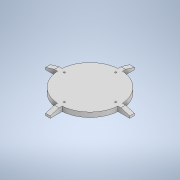
# Autodesk Inventor part: BASE
Saved by Autodesk Inventor 2021 (Build 250183000, 183)
## iProperties
Created: 2023-04-04
Part Number: BASE
Material: Generic
Document SubType Name: Modeling
Designer: PC
Density: 1 g/cm^3
Appearance: Default
Author: PC
Autodesk Inventor part; units mm, degrees
ref_plane "YZ Plane" through (0, 0, 0) normal (1, 0, 0) x (0, 1, 0)
ref_plane "XZ Plane" through (0, 0, 0) normal (0, 1, 0) x (-1, 0, 0)
ref_plane "XY Plane" through (0, 0, 0) normal (0, 0, 1) x (1, 0, 0)
ref_plane "Work Plane17" through (0, -15, 0) normal (0, -1, 0) x (1, 0, 0)
sketch "Sketch131" plane through (0, -15, 0) normal (0, -1, 0) x (1, 0, 0)
  circle A0 centre (0, 0) radius 2.55 projected
  circle A1 centre (0, 0) radius 65
  dimension "d245" = 130
  constraints: 1 centre point, 1 coincident
  measures "d245" diameter of A1
extrude "Extrusion62" add sketch "Sketch131" against normal blind 10 contours A0 | A1
sketch "Sketch132" plane through (0, -15, 0) normal (0, -1, 0) x (1, 0, 0)
  line L0 (5, 40) -> (-5, 40)
  line L1 (-5, 40) -> (-5, 90)
  line L2 (-5, 90) -> (5, 90)
  line L3 (5, 90) -> (5, 40)
  circle A0 centre (0, 0) radius 65 projected
  line L4 (5, 40) -> (-5, 90) construction
  line L5 (-5, 40) -> (5, 90) construction
  line L6 (-40, -5) -> (-90, -5)
  line L7 (-90, -5) -> (-90, 5)
  line L8 (-90, 5) -> (-40, 5)
  line L9 (-40, 5) -> (-40, -5)
  line L10 (-40, -5) -> (-90, 5) construction
  line L11 (-90, -5) -> (-40, 5) construction
  line L12 (5, -40) -> (-5, -40)
  line L13 (-5, -40) -> (-5, -90)
  line L14 (-5, -90) -> (5, -90)
  line L15 (5, -90) -> (5, -40)
  line L16 (5, -40) -> (-5, -90) construction
  line L17 (-5, -40) -> (5, -90) construction
  line L18 (89.9938, -5) -> (39.9938, -5)
  line L19 (39.9938, -5) -> (39.9938, 5)
  line L20 (39.9938, 5) -> (89.9938, 5)
  line L21 (89.9938, 5) -> (89.9938, -5)
  line L22 (89.9938, -5) -> (39.9938, 5) construction
  line L23 (39.9938, -5) -> (89.9938, 5) construction
  point P0 (0, 65)
  point P1 (-65, 0)
  point P2 (0, -65)
  point P3 (64.9938, 0)
  dimension "d248" = 10
  dimension "d249" = 50
  dimension "d250" = 50
  dimension "d251" = 10
  dimension "d252" = 10
  dimension "d253" = 50
  dimension "d254" = 50
  dimension "d255" = 10
  constraints: 48 end point, 8 midpoint, 8 parallel, 4 horizontal, 4 perpendicular, 3 point on circle
  measures "d248" distance of L1.end L2.end
  measures "d249" distance of L0.end L1.end
  measures "d250" distance of L7.end L8.end
  measures "d251" distance of L6.end L7.end
  measures "d252" distance of L14.end L13.end
  measures "d253" distance of L13.end L12.end
  measures "d254" distance of L19.end L20.end
  measures "d255" distance of L18.end L19.end
extrude "Extrusion63" add sketch "Sketch132" against normal blind 10 contours L0 L1 A0 L3 | A0 L1 L2 L3 | L20 L21 L18 A0 | A0 L18 L19 L20 | L8 L9 L6 A0 | A0 L6 L7 L8 | L13 L12 L15 A0 | A0 L15 L14 L13
chamfer "Chamfer1" distance 18.75 distance2 5.5 1 edges at (-90, -5, 0) measured on face at (-89.5, -5, 0)
chamfer "Chamfer2" distance 18.75 distance2 5.5 1 edges at (0, -5, -90) measured on face at (0, -5, -89.5)
chamfer "Chamfer3" distance 18.75 distance2 5.5 1 edges at (89.9938, -5, 0) measured on face at (89.4938, -5, 0)
chamfer "Chamfer4" distance 18.75 distance2 5.5 1 edges at (0, -5, 90) measured on face at (0, -5, 89.5)
sketch "Sketch135" plane through (0, -5, 0) normal (0, 1, 0) x (1, 0, 0)
  circle A0 centre (0, 0) radius 55.054
  circle A1 centre (-55.054, 0) radius 1.55
  circle A2 centre (0, 55.054) radius 1.55
  circle A3 centre (55.054, 0) radius 1.55
  circle A4 centre (0, -55.054) radius 1.55
  dimension "d279" = 110.108
  dimension "d280" = 3.1
  dimension "d281" = 3.1
  dimension "d282" = 3.1
  dimension "d283" = 3.1
  constraints: 5 centre point, 4 point on circle, 1 coincident
  measures "d279" diameter of A0
  measures "d280" diameter of A1
  measures "d281" diameter of A2
  measures "d282" diameter of A3
  measures "d283" diameter of A4
extrude "Extrusion64" cut sketch "Sketch135" against normal blind 30 contours A0 A3 | A0 A3 | A2 A0 | A0 A2 | A4 A0 | A0 A4 | A1 A0 | A0 A1
sketch "Sketch136" plane through (0, -15, 0) normal (0, -1, 0) x (1, 0, 0)
  circle A0 centre (-55.054, 0) radius 1.55 projected
  circle A1 centre (-55.054, 0) radius 4
  circle A2 centre (0, 55.054) radius 1.55 projected
  circle A3 centre (0, 55.054) radius 4
  circle A4 centre (55.054, 0) radius 1.55 projected
  circle A5 centre (55.054, 0) radius 4
  circle A6 centre (0, -55.054) radius 1.55 projected
  circle A7 centre (0, -55.054) radius 4
  point P0 (0, 0)
  dimension "d286" = 8
  dimension "d287" = 8
  dimension "d288" = 8
  dimension "d289" = 8
  constraints: 4 centre point, 4 coincident
  measures "d286" diameter of A1
  measures "d287" diameter of A3
  measures "d288" diameter of A5
  measures "d289" diameter of A7
extrude "Extrusion65" cut sketch "Sketch136" against normal blind 3.5 contours A0 | A1 | A2 | A3 | A4 | A5 | A6 | A7
body "Solid1"
